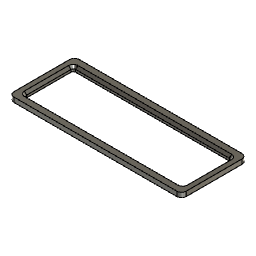
lcd top (Autodesk Fusion 360 design; units mm, degrees)
Autodesk Fusion 360 part; units mm, degrees
sketch "Sketch1" plane through (0, 0, 0) normal (0, 0, 1) x (1, 0, 0)
  line L0 (0, 0) -> (74, 0)
  line L1 (74, 0) -> (74, 28)
  line L2 (74, 28) -> (0, 28)
  line L3 (0, 28) -> (0, 0)
  dimension "d1" = 74
  dimension "d2" = 28
  constraint horizontal L0
  constraint vertical L1
  constraint horizontal L2
  constraint vertical L3
  constraint coincident L0.start L3.end
  measures "d1" distance of L0.start L0.end
  measures "d2" distance of L0 L2
extrude "Extrude1" add sketch "Sketch1" along normal blind 2
sketch "Sketch2" plane through (0, 0, 2) normal (0, 0, 1) x (-1, 0, 0)
  line L0 (0, -28) -> (0, 0)
  line L1 (0, 0) -> (-74, 0)
  line L2 (-74, 0) -> (-74, -28)
  line L3 (-74, -28) -> (0, -28)
  line L4 (-3, -24.5) -> (-71, -24.5)
  line L5 (-71, -24.5) -> (-71, -3.5)
  line L6 (-71, -3.5) -> (-3, -3.5)
  line L7 (-3, -3.5) -> (-3, -24.5)
  dimension "d5" = 3.5
  dimension "d6" = 3
  dimension "d7" = 3.5
  dimension "d8" = 3
  constraint horizontal L4
  constraint vertical L5
  constraint horizontal L6
  constraint vertical L7
  measures "d5" distance of L3 L4
  measures "d6" distance of L2 L5
  measures "d7" distance of L1 L6
  measures "d8" distance of L0 L7
extrude "Extrude2" cut sketch "Sketch2" against normal blind 2 contours L4 L5 L6 L7
fillet "Fillet1" radius 2 4 edges at (74, 0, 1) (74, 28, 1) (0, 28, 1) (0, 0, 1)
fillet "Fillet2" radius 1 4 edges at (71, 24.5, 1) (3, 24.5, 1) (3, 3.5, 1) (71, 3.5, 1)
chamfer "Chamfer1" distance 1 angle 45 8 edges at (3.2929, 3.7929, 2) (3, 14, 2) (3.2929, 24.2071, 2) (37, 24.5, 2) (70.7071, 24.2071, 2) (71, 14, 2) (70.7071, 3.7929, 2) (37, 3.5, 2)
